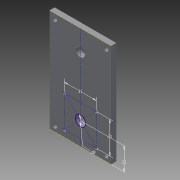
# Autodesk Inventor part: plate_bot
Saved by Autodesk Inventor 2015 SP2 (Build 190223200, 223)
## iProperties
Created: 2016-03-07
Part Number: plate_bot
Material: Generic
Document SubType Name: Modeling
Designer: marc
Density: 1 g/cm^3
Appearance: Default
Author: marc
Autodesk Inventor part; units mm, degrees
ref_plane "YZ Plane" through (0, 0, 0) normal (1, 0, 0) x (0, 1, 0)
ref_plane "XZ Plane" through (0, 0, 0) normal (0, 1, 0) x (-1, 0, 0)
ref_plane "XY Plane" through (0, 0, 0) normal (0, 0, 1) x (1, 0, 0)
sketch "Sketch1" plane through (0, 0, 0) normal (0, 1, 0) x (-1, 0, 0)
  line L0 (0, 0) -> (60, 0)
  line L1 (60, 0) -> (60, -100)
  line L2 (60, -100) -> (0, -100)
  line L3 (0, -100) -> (0, 0)
  dimension "d0" = 100
  dimension "d1" = 60
  constraints: 8 end point, 2 parallel, 1 horizontal, 1 perpendicular
  measures "d0" distance of L2.end L0.start
  measures "d1" distance between parallel lines of L1 L3
extrude "Extrusion1" add sketch "Sketch1" along normal blind 5
sketch "Sketch2" plane through (0, 0, 0) normal (0, -1, 0) x (1, 0, 0)
  line L0 (-60, 0) -> (0, 0) construction
  line L1 (-30, 0) -> (-30, -100) construction
  line L2 (0, -100) -> (-60, -100) construction
  line L3 (-14.5, -62.5) -> (-45.5, -62.5) construction
  line L4 (-45.5, -62.5) -> (-45.5, -93.5) construction
  line L5 (-45.5, -93.5) -> (-14.5, -93.5) construction
  line L6 (-14.5, -93.5) -> (-14.5, -62.5) construction
  line L7 (-14.5, -62.5) -> (-45.5, -93.5) construction
  line L8 (-45.5, -62.5) -> (-14.5, -93.5) construction
  circle A0 centre (-30, -78) radius 5
  point P0 (-30, -78)
  dimension "d7" = 31
  dimension "d8" = 31
  dimension "d9" = 22
  dimension "d25" = 10
  constraints: 14 end point, 5 coincident, 5 midpoint, 2 parallel, 1 centre point, 1 horizontal, 1 perpendicular, 1 point on line
  measures "d7" distance of L3.start L3.end
  measures "d8" distance of L5.end L3.start
  measures "d9" distance from line of L2 point (-30, -78)
  measures "d25" diameter of A0
hole "Hole1" at (-14.5, 0, -62.5) at (-14.5, 0, -93.5) at (-45.5, 0, -62.5) at (-45.5, 0, -93.5) direction (0, 1, 0) diameter 3.4 end through all clearance for "Socket Head Cap Screw ISO 4762" size "M3" standard "ISO"
sketch "Sketch3" plane through (0, 0, 0) normal (0, -1, 0) x (1, 0, 0)
  line L0 (-60, 0) -> (0, 0) construction
  line L1 (-30, 0) -> (-30, -100) construction
  line L2 (0, -100) -> (-60, -100) construction
  point P0 (-30, -20)
  dimension "d17" = 80
  constraints: 2 end point, 2 midpoint, 1 point on line
  measures "d17" distance from line of point (-30, -20) L2
hole "Hole2" at (-30, 0, -20) direction (0, 1, 0) diameter 9 end through all clearance for "Socket Head Cap Screw ISO 4762" size "M8" standard "ISO"
extrude "Extrusion2" cut sketch "Sketch2" against normal through all
sketch "Sketch4" plane through (0, 0, 0) normal (0, -1, 0) x (1, 0, 0)
  line L0 (0, -100) -> (0, 0) construction
  line L1 (0, -50) -> (-60, -50) construction
  line L2 (-60, 0) -> (-60, -100) construction
  line L3 (-55, -5) -> (-5, -5) construction
  line L4 (-5, -5) -> (-5, -95) construction
  line L5 (-5, -95) -> (-55, -95) construction
  line L6 (-55, -95) -> (-55, -5) construction
  line L7 (-55, -5) -> (-5, -95) construction
  line L8 (-5, -5) -> (-55, -95) construction
  line L9 (0, 0) -> (-60, 0) construction
  point P0 (-30, -50)
  point P1 (-30, -50)
  dimension "d28" = 5
  dimension "d29" = 5
  constraints: 14 end point, 7 midpoint, 4 coincident, 2 parallel, 1 horizontal, 1 perpendicular
  measures "d28" distance between parallel lines of L0 L4
  measures "d29" distance between parallel lines of L9 L3
hole "Hole3" at (-5, 0, -5) at (-55, 0, -5) at (-55, 0, -95) at (-5, 0, -95) direction (0, 1, 0) diameter 4.5 end through all clearance for "Socket Head Cap Screw ISO 4762" size "M4" standard "ISO"
body "Solid1"
